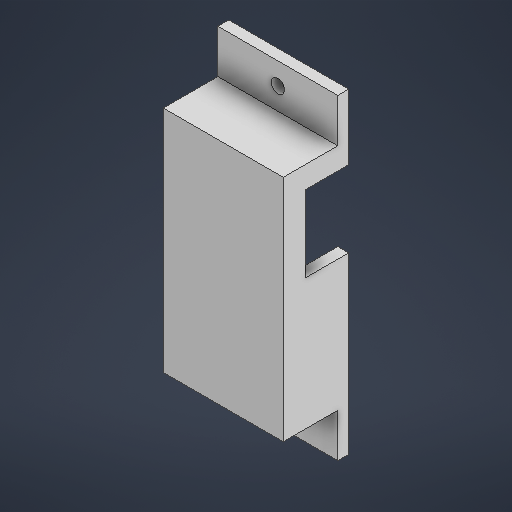
# Autodesk Inventor part: Hub
Saved by Autodesk Inventor 2026.2 (Build 302298000, 298)
## iProperties
Created: 2026-01-08
Part Number: Hub
Material: Generisch
Document SubType Name: Modeling
Designer: Alex
Density: 1 g/cm^3
Appearance: Vorgabe
Author: Alex
Autodesk Inventor part; units mm, degrees
ref_plane "YZ Plane" through (0, 0, 0) normal (1, 0, 0) x (0, 1, 0)
ref_plane "XZ Plane" through (0, 0, 0) normal (0, 1, 0) x (-1, 0, 0)
ref_plane "XY Plane" through (0, 0, 0) normal (0, 0, 1) x (1, 0, 0)
sketch "Skizze1" plane through (0, 0, 0) normal (0, 1, 0) x (-1, 0, 0)
  line L0 (-27.5, 52.5) -> (27.5, 52.5)
  line L1 (27.5, 52.5) -> (27.5, -52.5)
  line L2 (27.5, -52.5) -> (-27.5, -52.5)
  line L3 (-27.5, -52.5) -> (-27.5, 52.5)
  line L4 (-27.5, 52.5) -> (27.5, -52.5) construction
  line L5 (27.5, 52.5) -> (-27.5, -52.5) construction
  point P0 (0, 0)
  dimension "d0" = 55
  dimension "d1" = 105
  constraints: 12 end point, 2 midpoint, 2 parallel, 1 horizontal, 1 perpendicular
  measures "d0" distance of L1.end L2.end
  measures "d1" distance of L0.end L1.end
extrude "Extrusion1" add sketch "Skizze1" along normal blind 5
sketch "Skizze2" plane through (0, 5, 0) normal (0, 1, 0) x (1, 0, 0)
  line L0 (27.5, 52.5) -> (-27.5, 52.5) projected
  line L1 (-27.5, 52.5) -> (-27.5, -52.5) projected
  line L2 (-27.5, -52.5) -> (27.5, -52.5) projected
  line L3 (27.5, -52.5) -> (27.5, 52.5) projected
  line L4 (-27.5, -52.5) -> (27.5, -52.5)
  line L5 (27.5, -52.5) -> (27.5, -47.5)
  line L6 (27.5, -47.5) -> (-27.5, -47.5)
  line L7 (-27.5, -47.5) -> (-27.5, -52.5)
  line L8 (27.5, -47.5) -> (22.5, -47.5)
  line L9 (22.5, -47.5) -> (22.5, 52.5)
  line L10 (22.5, 52.5) -> (27.5, 52.5)
  line L11 (27.5, 52.5) -> (27.5, -47.5)
  line L12 (22.5, 52.5) -> (-27.5, 52.5)
  line L13 (-27.5, 52.5) -> (-27.5, 47.5)
  line L14 (-27.5, 47.5) -> (22.5, 47.5)
  line L15 (22.5, 47.5) -> (22.5, 52.5)
  point P0 (0, 0)
  dimension "d4" = 5
  dimension "d5" = 5
  dimension "d6" = 5
  constraints: 24 end point, 6 parallel, 3 horizontal, 3 perpendicular, 3 point on line
  measures "d4" distance of L5.end L4.end
  measures "d5" distance of L9.end L10.end
  measures "d6" distance of L13.end L12.end
extrude "Extrusion2" add sketch "Skizze2" along normal blind 25 contours L3 L6 L9 L0 | L9 L14 L1 L0 | L3 L2 L1 L6
sketch "Skizze3" plane through (27.5, 0, -52.5) normal (0, 0, -1) x (-1, 0, 0)
  line L0 (0, 0) -> (55, 0) projected
  line L1 (55, 0) -> (55, 30) projected
  line L2 (0, 30) -> (55, 30) projected
  line L3 (0, 0) -> (0, 30) projected
  line L4 (55, 30) -> (0, 30)
  line L5 (0, 30) -> (0, 25)
  line L6 (0, 25) -> (55, 25)
  line L7 (55, 25) -> (55, 30)
  point P0 (27.5, 0)
  dimension "d9" = 5
  constraints: 8 end point, 2 parallel, 1 horizontal, 1 perpendicular, 1 point on line
  measures "d9" distance of L5.end L4.end
extrude "Extrusion3" add sketch "Skizze3" along normal blind 20 contours L3 L2 L1 L6
sketch "Skizze4" plane through (-27.5, 0, 52.5) normal (0, 0, 1) x (1, 0, 0)
  line L0 (0, 0) -> (55, 0) projected
  line L1 (55, 0) -> (55, 30) projected
  line L2 (0, 30) -> (55, 30) projected
  line L3 (0, 0) -> (0, 30) projected
  line L4 (55, 25) -> (0, 25) projected
  line L5 (0, 30) -> (55, 30)
  line L6 (55, 30) -> (55, 25)
  line L7 (55, 25) -> (0, 25)
  line L8 (0, 25) -> (0, 30)
  point P0 (27.5, 0)
  dimension "d12" = 5
  constraints: 8 end point, 2 parallel, 1 horizontal, 1 perpendicular
  measures "d12" distance of L5.end L4.start
extrude "Extrusion4" add sketch "Skizze4" along normal blind 20 contours L3 L2 L1 L4
sketch "Skizze5" plane through (0, 30, 0) normal (0, 1, 0) x (1, 0, 0)
  line L0 (-27.5, -47.5) -> (-27.5, -72.5) projected
  line L1 (27.5, -72.5) -> (-27.5, -72.5) projected
  line L2 (27.5, 72.5) -> (27.5, -72.5) projected
  line L3 (-27.5, 72.5) -> (27.5, 72.5) projected
  line L4 (-27.5, 47.5) -> (-27.5, 72.5) projected
  line L5 (-27.5, 47.5) -> (22.5, 47.5) projected
  line L6 (22.5, 47.5) -> (22.5, -47.5) projected
  line L7 (22.5, -47.5) -> (-27.5, -47.5) projected
  line L8 (0, 72.5) -> (0, 62.5)
  circle A0 centre (0, 62.5) radius 3.1
  line L9 (0, -72.5) -> (0, -62.5)
  circle A1 centre (0, -62.5) radius 3.1
  point P0 (0, 0)
  dimension "d15" = 10
  dimension "d16" = 6.2
  dimension "d17" = 10
  dimension "d18" = 6.2
  constraints: 4 end point, 2 centre point, 2 coincident, 2 midpoint, 2 vertical
  measures "d15" distance of L8.start L8.end
  measures "d16" diameter of A0
  measures "d17" distance of L9.start L9.end
  measures "d18" diameter of A1
extrude "Extrusion5" cut sketch "Skizze5" against normal blind 20 contours A1 | A0
sketch "Skizze6" plane through (0, 30, 0) normal (0, 1, 0) x (1, 0, 0)
  circle A0 centre (0, 62.5) radius 3.1 projected
  circle A1 centre (0, -62.5) radius 3.1 projected
  line L0 (-27.5, -47.5) -> (-27.5, -72.5) projected
  line L1 (27.5, -72.5) -> (-27.5, -72.5) projected
  line L2 (27.5, 72.5) -> (27.5, -72.5) projected
  line L3 (-27.5, 72.5) -> (27.5, 72.5) projected
  line L4 (-27.5, 47.5) -> (-27.5, 72.5) projected
  line L5 (-27.5, 47.5) -> (22.5, 47.5) projected
  line L6 (22.5, 47.5) -> (22.5, -47.5) projected
  line L7 (22.5, -47.5) -> (-27.5, -47.5) projected
  line L8 (22.5, -47.5) -> (27.5, -47.5)
  line L9 (22.5, -47.5) -> (22.5, -42.5)
  line L10 (22.5, -42.5) -> (27.5, -42.5)
  line L11 (22.5, -42.5) -> (22.5, -7.5)
  line L12 (22.5, 47.5) -> (22.5, -47.5) projected
  line L13 (22.5, -7.5) -> (27.5, -7.5)
  point P0 (0, 0)
  dimension "d21" = 5
  dimension "d22" = 35
  constraints: 10 end point, 5 point on line, 3 perpendicular
  measures "d21" distance of L6.end L9.end
  measures "d22" distance of L9.end L11.end
extrude "Extrusion6" cut sketch "Skizze6" against normal blind 20 contours L6 L13 L2 L10
